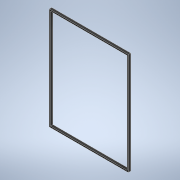
# Autodesk Inventor part: rubberSeal
Saved by Autodesk Inventor 2022.6 (Build 266554010, 554A)
## iProperties
Created: 2025-03-20
Part Number: rubberSeal
Material: Generic
Document SubType Name: Modeling
Designer: khinm
Density: 1 g/cm^3
Appearance: Rubber - Black
Author: khinm
Autodesk Inventor part; units mm, degrees
ref_plane "YZ Plane" through (0, 0, 0) normal (1, 0, 0) x (0, 1, 0)
ref_plane "XZ Plane" through (0, 0, 0) normal (0, 1, 0) x (-1, 0, 0)
ref_plane "XY Plane" through (0, 0, 0) normal (0, 0, 1) x (1, 0, 0)
sketch "Sketch1" plane through (0, 0, 0) normal (0, 0, 1) x (1, 0, 0)
  line L0 (0, 0) -> (155, 0)
  line L1 (155, 0) -> (155, 200)
  line L2 (155, 200) -> (0, 200)
  line L3 (0, 200) -> (0, 0)
  dimension "d0" = 200
  dimension "d1" = 155
  constraints: 8 end point, 2 parallel, 1 coincident, 1 horizontal, 1 perpendicular
  measures "d0" distance of L0.end L1.end
  measures "d1" distance of L1.end L2.end
extrude "Extrusion1" add sketch "Sketch1" along normal blind 5
sketch "Sketch2" plane through (0, 0, 5) normal (0, 0, 1) x (1, 0, 0)
  line L0 (155, 0) -> (155, 200) projected
  line L1 (155, 200) -> (0, 200) projected
  line L2 (0, 200) -> (0, 0) projected
  line L3 (0, 0) -> (155, 0) projected
  line L4 (2.5, 197.5) -> (152.5, 197.5)
  line L5 (152.5, 197.5) -> (152.5, 2.5)
  line L6 (152.5, 2.5) -> (2.5, 2.5)
  line L7 (2.5, 2.5) -> (2.5, 197.5)
  dimension "d4" = 150
  dimension "d5" = 195
  dimension "d6" = 2.5
  dimension "d7" = 2.5
  constraints: 8 end point, 2 parallel, 1 horizontal, 1 perpendicular
  measures "d4" distance of L5.end L6.end
  measures "d5" distance between parallel lines of L6 L4
  measures "d6" distance between parallel lines of L3 L6
  measures "d7" distance between parallel lines of L2 L7
extrude "Extrusion2" cut sketch "Sketch2" against normal up to surface (5 mm away) contours L4 L5 L6 L7
body "Solid1"
